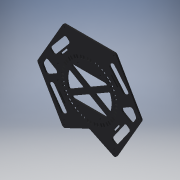
# Autodesk Inventor part: Bottom Plate
Saved by Autodesk Inventor 2017 (Build 210142000, 142)
## iProperties
Created: 2016-10-01
Part Number: Bottom Plate
Material: PVC, Unplasticized
Document SubType Name: Modeling
Designer: James Yelland
Density: 1.29 g/cm^3
Appearance: Smooth - White
Mass: 43.6601 g
Surface Area: 401.333 cm^2
Volume: 33.8451 cm^3
Author: James Yelland
Autodesk Inventor part; units mm, degrees
ref_plane "YZ Plane" through (0, 0, 0) normal (1, 0, 0) x (0, 1, 0)
ref_plane "XZ Plane" through (0, 0, 0) normal (0, 1, 0) x (-1, 0, 0)
ref_plane "XY Plane" through (0, 0, 0) normal (0, 0, 1) x (1, 0, 0)
sketch "Sketch1" plane through (0, 0, 0) normal (0, 1, 0) x (-1, 0, 0)
  line L0 (103.5566, -2.5) -> (54.8095, -86.9325)
  line L1 (-54.8095, -86.9325) -> (-103.5566, -2.5)
  line L2 (-103.5566, 2.5) -> (-53.9434, 88.4327)
  line L3 (-49.6132, 90.9327) -> (49.6132, 90.9327)
  line L4 (53.9434, 88.4327) -> (103.5566, 2.5)
  line L5 (2.1497, -66.9563) -> (48.3297, -88.9468)
  line L6 (-2.1497, -66.9563) -> (-48.3297, -88.9468)
  arc A0 (48.3297, -88.9468) -> (54.8095, -86.9325) centre (50.4794, -84.4325) ccw
  arc A1 (2.1497, -66.9563) -> (-2.1497, -66.9563) centre (0, -71.4706) ccw
  arc A2 (-54.8095, -86.9325) -> (-48.3297, -88.9468) centre (-50.4794, -84.4325) ccw
  arc A3 (-103.5566, 2.5) -> (-103.5566, -2.5) centre (-99.2265, 0) ccw
  arc A4 (-49.6132, 90.9327) -> (-53.9434, 88.4327) centre (-49.6132, 85.9327) ccw
  arc A5 (53.9434, 88.4327) -> (49.6132, 90.9327) centre (49.6132, 85.9327) ccw
  arc A6 (103.5566, -2.5) -> (103.5566, 2.5) centre (99.2265, 0) ccw
  circle A7 centre (49.6132, 85.9327) radius 1.6
  circle A8 centre (-49.6132, 85.9327) radius 1.6
  circle A9 centre (-99.2265, 0) radius 1.6
  circle A10 centre (99.2265, 0) radius 1.6
  arc A11 (-88.75, -10.8253) -> (-81.9199, -12.6554) centre (-84.4199, -8.3253) ccw
  arc A12 (-93.5566, 2.5) -> (-93.5566, -2.5) centre (-89.2265, 0) ccw
  arc A13 (81.9199, -12.6554) -> (88.75, -10.8253) centre (84.4199, -8.3253) ccw
  arc A14 (93.5566, -2.5) -> (93.5566, 2.5) centre (89.2265, 0) ccw
  line L7 (1.5, -53.75) -> (1.5, -56.75)
  line L8 (1.5, -56.75) -> (4.5, -56.75)
  line L9 (4.5, -56.75) -> (4.5, -50.75)
  line L10 (4.5, -50.75) -> (1.5, -50.75)
  line L11 (1.5, -50.75) -> (1.5, -53.75)
  line L12 (-1.5, -53.75) -> (-1.5, -56.75)
  line L13 (-1.5, -56.75) -> (-4.5, -56.75)
  line L14 (-1.5, -53.75) -> (-1.5, -53.75)
  line L15 (-1.5, -53.75) -> (-1.5, -50.75)
  line L16 (-1.5, -50.75) -> (-4.5, -50.75)
  line L17 (-4.5, -56.75) -> (-4.5, -50.75)
  line L18 (15.3604, -51.5303) -> (16.1369, -54.4281)
  line L19 (16.1369, -54.4281) -> (19.0346, -53.6516)
  line L20 (19.0346, -53.6516) -> (17.4817, -47.856)
  line L21 (17.4817, -47.856) -> (14.584, -48.6325)
  line L22 (14.584, -48.6325) -> (15.3604, -51.5303)
  line L23 (12.4626, -52.3067) -> (13.2391, -55.2045)
  line L24 (13.2391, -55.2045) -> (10.3413, -55.981)
  line L25 (12.4626, -52.3067) -> (11.6862, -49.409)
  line L26 (11.6862, -49.409) -> (8.7884, -50.1854)
  line L27 (10.3413, -55.981) -> (8.7884, -50.1854)
  line L28 (28.174, -45.7989) -> (29.674, -48.3969)
  line L29 (29.674, -48.3969) -> (32.2721, -46.8969)
  line L30 (32.2721, -46.8969) -> (29.2721, -41.7008)
  line L31 (29.2721, -41.7008) -> (26.674, -43.2008)
  line L32 (26.674, -43.2008) -> (28.174, -45.7989)
  line L33 (25.576, -47.2989) -> (27.076, -49.8969)
  line L34 (27.076, -49.8969) -> (24.4779, -51.3969)
  line L35 (25.576, -47.2989) -> (24.076, -44.7008)
  line L36 (24.076, -44.7008) -> (21.4779, -46.2008)
  line L37 (24.4779, -51.3969) -> (21.4779, -46.2008)
  line L38 (39.0676, -36.9463) -> (41.189, -39.0676)
  line L39 (41.189, -39.0676) -> (43.3103, -36.9463)
  line L40 (43.3103, -36.9463) -> (39.0676, -32.7037)
  line L41 (39.0676, -32.7037) -> (36.9463, -34.825)
  line L42 (36.9463, -34.825) -> (39.0676, -36.9463)
  line L43 (36.9463, -39.0676) -> (39.0676, -41.189)
  line L44 (39.0676, -41.189) -> (36.9463, -43.3103)
  line L45 (36.9463, -39.0676) -> (34.825, -36.9463)
  line L46 (34.825, -36.9463) -> (32.7037, -39.0676)
  line L47 (36.9463, -43.3103) -> (32.7037, -39.0676)
  line L48 (47.2989, -25.576) -> (49.8969, -27.076)
  line L49 (49.8969, -27.076) -> (51.3969, -24.4779)
  line L50 (51.3969, -24.4779) -> (46.2008, -21.4779)
  line L51 (46.2008, -21.4779) -> (44.7008, -24.076)
  line L52 (44.7008, -24.076) -> (47.2989, -25.576)
  line L53 (45.7989, -28.174) -> (48.3969, -29.674)
  line L54 (48.3969, -29.674) -> (46.8969, -32.2721)
  line L55 (45.7989, -28.174) -> (43.2008, -26.674)
  line L56 (43.2008, -26.674) -> (41.7008, -29.2721)
  line L57 (46.8969, -32.2721) -> (41.7008, -29.2721)
  line L58 (52.3067, -12.4626) -> (55.2045, -13.2391)
  line L59 (55.2045, -13.2391) -> (55.981, -10.3413)
  line L60 (55.981, -10.3413) -> (50.1854, -8.7884)
  line L61 (50.1854, -8.7884) -> (49.409, -11.6862)
  line L62 (49.409, -11.6862) -> (52.3067, -12.4626)
  line L63 (51.5303, -15.3604) -> (54.4281, -16.1369)
  line L64 (54.4281, -16.1369) -> (53.6516, -19.0346)
  line L65 (51.5303, -15.3604) -> (48.6325, -14.584)
  line L66 (48.6325, -14.584) -> (47.856, -17.4817)
  line L67 (53.6516, -19.0346) -> (47.856, -17.4817)
  line L68 (53.75, 1.5) -> (56.75, 1.5)
  line L69 (56.75, 1.5) -> (56.75, 4.5)
  line L70 (56.75, 4.5) -> (50.75, 4.5)
  line L71 (50.75, 4.5) -> (50.75, 1.5)
  line L72 (50.75, 1.5) -> (53.75, 1.5)
  line L73 (53.75, -1.5) -> (56.75, -1.5)
  line L74 (56.75, -1.5) -> (56.75, -4.5)
  line L75 (53.75, -1.5) -> (50.75, -1.5)
  line L76 (50.75, -1.5) -> (50.75, -4.5)
  line L77 (56.75, -4.5) -> (50.75, -4.5)
  line L78 (51.5303, 15.3604) -> (54.4281, 16.1369)
  line L79 (54.4281, 16.1369) -> (53.6516, 19.0346)
  line L80 (53.6516, 19.0346) -> (47.856, 17.4817)
  line L81 (47.856, 17.4817) -> (48.6325, 14.584)
  line L82 (48.6325, 14.584) -> (51.5303, 15.3604)
  line L83 (52.3067, 12.4626) -> (55.2045, 13.2391)
  line L84 (55.2045, 13.2391) -> (55.981, 10.3413)
  line L85 (52.3067, 12.4626) -> (49.409, 11.6862)
  line L86 (49.409, 11.6862) -> (50.1854, 8.7884)
  line L87 (55.981, 10.3413) -> (50.1854, 8.7884)
  line L88 (45.7989, 28.174) -> (48.3969, 29.674)
  line L89 (48.3969, 29.674) -> (46.8969, 32.2721)
  line L90 (46.8969, 32.2721) -> (41.7008, 29.2721)
  line L91 (41.7008, 29.2721) -> (43.2008, 26.674)
  line L92 (43.2008, 26.674) -> (45.7989, 28.174)
  line L93 (47.2989, 25.576) -> (49.8969, 27.076)
  line L94 (49.8969, 27.076) -> (51.3969, 24.4779)
  line L95 (47.2989, 25.576) -> (44.7008, 24.076)
  line L96 (44.7008, 24.076) -> (46.2008, 21.4779)
  line L97 (51.3969, 24.4779) -> (46.2008, 21.4779)
  line L98 (36.9463, 39.0676) -> (39.0676, 41.189)
  line L99 (39.0676, 41.189) -> (36.9463, 43.3103)
  line L100 (36.9463, 43.3103) -> (32.7037, 39.0676)
  line L101 (32.7037, 39.0676) -> (34.825, 36.9463)
  line L102 (34.825, 36.9463) -> (36.9463, 39.0676)
  line L103 (39.0676, 36.9463) -> (41.189, 39.0676)
  line L104 (41.189, 39.0676) -> (43.3103, 36.9463)
  line L105 (39.0676, 36.9463) -> (36.9463, 34.825)
  line L106 (36.9463, 34.825) -> (39.0676, 32.7037)
  line L107 (43.3103, 36.9463) -> (39.0676, 32.7037)
  line L108 (25.576, 47.2989) -> (27.076, 49.8969)
  line L109 (27.076, 49.8969) -> (24.4779, 51.3969)
  line L110 (24.4779, 51.3969) -> (21.4779, 46.2008)
  line L111 (21.4779, 46.2008) -> (24.076, 44.7008)
  line L112 (24.076, 44.7008) -> (25.576, 47.2989)
  line L113 (28.174, 45.7989) -> (29.674, 48.3969)
  line L114 (29.674, 48.3969) -> (32.2721, 46.8969)
  line L115 (28.174, 45.7989) -> (26.674, 43.2008)
  line L116 (26.674, 43.2008) -> (29.2721, 41.7008)
  line L117 (32.2721, 46.8969) -> (29.2721, 41.7008)
  line L118 (12.4626, 52.3067) -> (13.2391, 55.2045)
  line L119 (13.2391, 55.2045) -> (10.3413, 55.981)
  line L120 (10.3413, 55.981) -> (8.7884, 50.1854)
  line L121 (8.7884, 50.1854) -> (11.6862, 49.409)
  line L122 (11.6862, 49.409) -> (12.4626, 52.3067)
  line L123 (15.3604, 51.5303) -> (16.1369, 54.4281)
  line L124 (16.1369, 54.4281) -> (19.0346, 53.6516)
  line L125 (15.3604, 51.5303) -> (14.584, 48.6325)
  line L126 (14.584, 48.6325) -> (17.4817, 47.856)
  line L127 (19.0346, 53.6516) -> (17.4817, 47.856)
  line L128 (-1.5, 53.75) -> (-1.5, 56.75)
  line L129 (-1.5, 56.75) -> (-4.5, 56.75)
  line L130 (-4.5, 56.75) -> (-4.5, 50.75)
  line L131 (-4.5, 50.75) -> (-1.5, 50.75)
  line L132 (-1.5, 50.75) -> (-1.5, 53.75)
  line L133 (1.5, 53.75) -> (1.5, 56.75)
  line L134 (1.5, 56.75) -> (4.5, 56.75)
  line L135 (1.5, 53.75) -> (1.5, 50.75)
  line L136 (1.5, 50.75) -> (4.5, 50.75)
  line L137 (4.5, 56.75) -> (4.5, 50.75)
  line L138 (-15.3604, 51.5303) -> (-16.1369, 54.4281)
  line L139 (-16.1369, 54.4281) -> (-19.0346, 53.6516)
  line L140 (-19.0346, 53.6516) -> (-17.4817, 47.856)
  line L141 (-17.4817, 47.856) -> (-14.584, 48.6325)
  line L142 (-14.584, 48.6325) -> (-15.3604, 51.5303)
  line L143 (-12.4626, 52.3067) -> (-13.2391, 55.2045)
  line L144 (-13.2391, 55.2045) -> (-10.3413, 55.981)
  line L145 (-12.4626, 52.3067) -> (-11.6862, 49.409)
  line L146 (-11.6862, 49.409) -> (-8.7884, 50.1854)
  line L147 (-10.3413, 55.981) -> (-8.7884, 50.1854)
  line L148 (-28.174, 45.7989) -> (-29.674, 48.3969)
  line L149 (-29.674, 48.3969) -> (-32.2721, 46.8969)
  line L150 (-32.2721, 46.8969) -> (-29.2721, 41.7008)
  line L151 (-29.2721, 41.7008) -> (-26.674, 43.2008)
  line L152 (-26.674, 43.2008) -> (-28.174, 45.7989)
  line L153 (-25.576, 47.2989) -> (-27.076, 49.8969)
  line L154 (-27.076, 49.8969) -> (-24.4779, 51.3969)
  line L155 (-25.576, 47.2989) -> (-24.076, 44.7008)
  line L156 (-24.076, 44.7008) -> (-21.4779, 46.2008)
  line L157 (-24.4779, 51.3969) -> (-21.4779, 46.2008)
  line L158 (-39.0676, 36.9463) -> (-41.189, 39.0676)
  line L159 (-41.189, 39.0676) -> (-43.3103, 36.9463)
  line L160 (-43.3103, 36.9463) -> (-39.0676, 32.7037)
  line L161 (-39.0676, 32.7037) -> (-36.9463, 34.825)
  line L162 (-36.9463, 34.825) -> (-39.0676, 36.9463)
  line L163 (-36.9463, 39.0676) -> (-39.0676, 41.189)
  line L164 (-39.0676, 41.189) -> (-36.9463, 43.3103)
  line L165 (-36.9463, 39.0676) -> (-34.825, 36.9463)
  line L166 (-34.825, 36.9463) -> (-32.7037, 39.0676)
  line L167 (-36.9463, 43.3103) -> (-32.7037, 39.0676)
  line L168 (-47.2989, 25.576) -> (-49.8969, 27.076)
  line L169 (-49.8969, 27.076) -> (-51.3969, 24.4779)
  line L170 (-51.3969, 24.4779) -> (-46.2008, 21.4779)
  line L171 (-46.2008, 21.4779) -> (-44.7008, 24.076)
  line L172 (-44.7008, 24.076) -> (-47.2989, 25.576)
  line L173 (-45.7989, 28.174) -> (-48.3969, 29.674)
  line L174 (-48.3969, 29.674) -> (-46.8969, 32.2721)
  line L175 (-45.7989, 28.174) -> (-43.2008, 26.674)
  line L176 (-43.2008, 26.674) -> (-41.7008, 29.2721)
  line L177 (-46.8969, 32.2721) -> (-41.7008, 29.2721)
  line L178 (-52.3067, 12.4626) -> (-55.2045, 13.2391)
  line L179 (-55.2045, 13.2391) -> (-55.981, 10.3413)
  line L180 (-55.981, 10.3413) -> (-50.1854, 8.7884)
  line L181 (-50.1854, 8.7884) -> (-49.409, 11.6862)
  line L182 (-49.409, 11.6862) -> (-52.3067, 12.4626)
  line L183 (-51.5303, 15.3604) -> (-54.4281, 16.1369)
  line L184 (-54.4281, 16.1369) -> (-53.6516, 19.0346)
  line L185 (-51.5303, 15.3604) -> (-48.6325, 14.584)
  line L186 (-48.6325, 14.584) -> (-47.856, 17.4817)
  line L187 (-53.6516, 19.0346) -> (-47.856, 17.4817)
  line L188 (-53.75, -1.5) -> (-56.75, -1.5)
  line L189 (-56.75, -1.5) -> (-56.75, -4.5)
  line L190 (-56.75, -4.5) -> (-50.75, -4.5)
  line L191 (-50.75, -4.5) -> (-50.75, -1.5)
  line L192 (-50.75, -1.5) -> (-53.75, -1.5)
  line L193 (-53.75, 1.5) -> (-56.75, 1.5)
  line L194 (-56.75, 1.5) -> (-56.75, 4.5)
  line L195 (-53.75, 1.5) -> (-50.75, 1.5)
  line L196 (-50.75, 1.5) -> (-50.75, 4.5)
  line L197 (-56.75, 4.5) -> (-50.75, 4.5)
  line L198 (-51.5303, -15.3604) -> (-54.4281, -16.1369)
  line L199 (-54.4281, -16.1369) -> (-53.6516, -19.0346)
  line L200 (-53.6516, -19.0346) -> (-47.856, -17.4817)
  line L201 (-47.856, -17.4817) -> (-48.6325, -14.584)
  line L202 (-48.6325, -14.584) -> (-51.5303, -15.3604)
  line L203 (-52.3067, -12.4626) -> (-55.2045, -13.2391)
  line L204 (-55.2045, -13.2391) -> (-55.981, -10.3413)
  line L205 (-52.3067, -12.4626) -> (-49.409, -11.6862)
  line L206 (-49.409, -11.6862) -> (-50.1854, -8.7884)
  line L207 (-55.981, -10.3413) -> (-50.1854, -8.7884)
  line L208 (-45.7989, -28.174) -> (-48.3969, -29.674)
  line L209 (-48.3969, -29.674) -> (-46.8969, -32.2721)
  line L210 (-46.8969, -32.2721) -> (-41.7008, -29.2721)
  line L211 (-41.7008, -29.2721) -> (-43.2008, -26.674)
  line L212 (-43.2008, -26.674) -> (-45.7989, -28.174)
  line L213 (-47.2989, -25.576) -> (-49.8969, -27.076)
  line L214 (-49.8969, -27.076) -> (-51.3969, -24.4779)
  line L215 (-47.2989, -25.576) -> (-44.7008, -24.076)
  line L216 (-44.7008, -24.076) -> (-46.2008, -21.4779)
  line L217 (-51.3969, -24.4779) -> (-46.2008, -21.4779)
  line L218 (-36.9463, -39.0676) -> (-39.0676, -41.189)
  line L219 (-39.0676, -41.189) -> (-36.9463, -43.3103)
  line L220 (-36.9463, -43.3103) -> (-32.7037, -39.0676)
  line L221 (-32.7037, -39.0676) -> (-34.825, -36.9463)
  line L222 (-34.825, -36.9463) -> (-36.9463, -39.0676)
  line L223 (-39.0676, -36.9463) -> (-41.189, -39.0676)
  line L224 (-41.189, -39.0676) -> (-43.3103, -36.9463)
  line L225 (-39.0676, -36.9463) -> (-36.9463, -34.825)
  line L226 (-36.9463, -34.825) -> (-39.0676, -32.7037)
  line L227 (-43.3103, -36.9463) -> (-39.0676, -32.7037)
  line L228 (-25.576, -47.2989) -> (-27.076, -49.8969)
  line L229 (-27.076, -49.8969) -> (-24.4779, -51.3969)
  line L230 (-24.4779, -51.3969) -> (-21.4779, -46.2008)
  line L231 (-21.4779, -46.2008) -> (-24.076, -44.7008)
  line L232 (-24.076, -44.7008) -> (-25.576, -47.2989)
  line L233 (-28.174, -45.7989) -> (-29.674, -48.3969)
  line L234 (-29.674, -48.3969) -> (-32.2721, -46.8969)
  line L235 (-28.174, -45.7989) -> (-26.674, -43.2008)
  line L236 (-26.674, -43.2008) -> (-29.2721, -41.7008)
  line L237 (-32.2721, -46.8969) -> (-29.2721, -41.7008)
  line L238 (-12.4626, -52.3067) -> (-13.2391, -55.2045)
  line L239 (-13.2391, -55.2045) -> (-10.3413, -55.981)
  line L240 (-10.3413, -55.981) -> (-8.7884, -50.1854)
  line L241 (-8.7884, -50.1854) -> (-11.6862, -49.409)
  line L242 (-11.6862, -49.409) -> (-12.4626, -52.3067)
  line L243 (-15.3604, -51.5303) -> (-16.1369, -54.4281)
  line L244 (-16.1369, -54.4281) -> (-19.0346, -53.6516)
  line L245 (-15.3604, -51.5303) -> (-14.584, -48.6325)
  line L246 (-14.584, -48.6325) -> (-17.4817, -47.856)
  line L247 (-19.0346, -53.6516) -> (-17.4817, -47.856)
  arc A15 (-81.9199, 12.6554) -> (-88.75, 10.8253) centre (-84.4199, 8.3253) ccw
  arc A16 (50.7976, 70.0378) -> (45.1623, 70.5308) centre (47.7335, 67.4666) ccw
  line L248 (45.1623, 70.5308) -> (41.3321, 67.3169)
  arc A17 (41.3321, 67.3169) -> (40.8391, 61.6815) centre (43.9032, 64.2527) ccw
  line L249 (64.2962, 53.9509) -> (50.7976, 70.0378)
  line L250 (40.8391, 61.6815) -> (67.8361, 29.5077)
  line L251 (64.2962, 53.9509) -> (77.7947, 37.8639)
  arc A18 (77.3017, 32.2286) -> (77.7947, 37.8639) centre (74.7305, 35.2928) ccw
  line L252 (73.4714, 29.0147) -> (77.3017, 32.2286)
  arc A19 (67.8361, 29.5077) -> (73.4714, 29.0147) centre (70.9003, 32.0789) ccw
  arc A20 (88.75, 10.8253) -> (81.9199, 12.6554) centre (84.4199, 8.3253) ccw
  arc A21 (67.5, 4.3301) -> (67.5, -4.3301) centre (70, 0) ccw
  arc A22 (-67.5, -4.3301) -> (-67.5, 4.3301) centre (-70, 0) ccw
  line L253 (-67.5, -4.3301) -> (-81.9199, -12.6554)
  line L254 (-88.75, -10.8253) -> (-93.5566, -2.5)
  line L255 (-93.5566, 2.5) -> (-88.75, 10.8253)
  line L256 (-81.9199, 12.6554) -> (-67.5, 4.3301)
  line L257 (81.9199, 12.6554) -> (67.5, 4.3301)
  line L258 (67.5, -4.3301) -> (81.9199, -12.6554)
  line L259 (88.75, -10.8253) -> (93.5566, -2.5)
  line L260 (93.5566, 2.5) -> (88.75, 10.8253)
  line L261 (0, 30) -> (-31.225, 30)
  line L262 (0, 30) -> (31.225, 30)
  line L263 (0, -30) -> (-31.225, -30)
  line L264 (0, -30) -> (31.225, -30)
  arc A23 (42.1141, -15.8557) -> (42.1141, 15.8557) centre (0, 0) ccw
  arc A24 (-42.1141, 15.8558) -> (-42.1141, -15.8558) centre (0, 0) ccw
  arc A25 (34.525, 28.7563) -> (31.225, 30) centre (31.225, 25) ccw
  arc A26 (-31.225, 30) -> (-34.525, 28.7563) centre (-31.225, 25) ccw
  arc A27 (-34.525, -28.7563) -> (-31.225, -30) centre (-31.225, -25) ccw
  arc A28 (31.225, -30) -> (34.525, -28.7563) centre (31.225, -25) ccw
  circle A29 centre (22.6343, 38) radius 1.6
  circle A30 centre (-22.6343, 38) radius 1.6
  circle A31 centre (-22.6343, -38) radius 1.6
  circle A32 centre (22.6343, -38) radius 1.6
  line L265 (54.3376, 45.5946) -> (57.5515, 41.7644)
  line L266 (39.2424, -16.8831) -> (13, -1.7321)
  line L267 (39.2424, 16.8831) -> (13, 1.7321)
  line L268 (34.205, 25.5218) -> (1, 6.3509)
  line L269 (-1, 6.3509) -> (-34.205, 25.5218)
  line L270 (-39.2423, 16.8832) -> (-12.9998, 1.7321)
  line L271 (-12.9998, -1.7321) -> (-39.2423, -16.8832)
  line L272 (-34.205, -25.5218) -> (-1, -6.3509)
  line L273 (1, -6.3509) -> (34.205, -25.5218)
  arc A33 (-1, 6.3509) -> (1, 6.3509) centre (0, 8.0829) ccw
  arc A34 (-12.9998, -1.7321) -> (-12.9998, 1.7321) centre (-13.9998, 0) ccw
  arc A35 (1, -6.3509) -> (-1, -6.3509) centre (0, -8.0829) ccw
  arc A36 (13, 1.7321) -> (13, -1.7321) centre (14, 0) ccw
  arc A37 (39.2424, -16.8831) -> (42.1141, -15.8557) centre (40.2424, -15.151) ccw
  arc A38 (34.525, -28.7563) -> (34.205, -25.5218) centre (33.205, -27.2538) ccw
  arc A39 (-42.1141, -15.8558) -> (-39.2423, -16.8832) centre (-40.2423, -15.1511) ccw
  arc A40 (-34.205, -25.5218) -> (-34.525, -28.7563) centre (-33.205, -27.2538) ccw
  arc A41 (-39.2423, 16.8832) -> (-42.1141, 15.8558) centre (-40.2423, 15.1511) ccw
  arc A42 (-34.525, 28.7563) -> (-34.205, 25.5218) centre (-33.205, 27.2538) ccw
  arc A43 (42.1141, 15.8557) -> (39.2424, 16.8831) centre (40.2424, 15.151) ccw
  arc A44 (34.205, 25.5218) -> (34.525, 28.7563) centre (33.205, 27.2538) ccw
  circle A45 centre (50.4794, -84.4325) radius 1.45
  circle A46 centre (50.4794, -76.4325) radius 1.45
  circle A47 centre (-50.4794, -84.4325) radius 1.45
  circle A48 centre (-50.4794, -76.4325) radius 1.45
  line L274 (49.7796, 41.77) -> (43.3517, 49.4305)
  line L275 (43.3517, 49.4305) -> (45.6499, 51.3589)
  line L276 (45.6499, 51.3589) -> (58.5056, 36.038)
  line L277 (58.5056, 36.038) -> (56.2075, 34.1096)
  line L278 (56.2075, 34.1096) -> (49.7796, 41.77)
  arc A49 (75.7207, -22.5008) -> (70.1497, -23.4831) centre (73.4264, -25.7774) ccw
  arc A50 (80.7987, -30.9396) -> (79.8164, -25.3687) centre (77.5221, -28.6453) ccw
  line L279 (75.7207, -22.5008) -> (79.8164, -25.3687)
  arc A51 (51.1376, -66.3263) -> (56.7085, -65.344) centre (53.4319, -63.0497) ccw
  line L280 (51.1376, -66.3263) -> (47.0419, -63.4584)
  arc A52 (46.0596, -57.8875) -> (47.0419, -63.4584) centre (49.3362, -60.1818) ccw
  line L281 (68.7536, -48.1418) -> (56.7085, -65.344)
  line L282 (68.7536, -48.1418) -> (80.7987, -30.9396)
  line L283 (46.0596, -57.8875) -> (70.1497, -23.4831)
  line L284 (58.1046, -40.6853) -> (60.9725, -36.5895)
  line L285 (53.2307, -37.2725) -> (47.4949, -45.464)
  line L286 (47.4949, -45.464) -> (49.9524, -47.1848)
  line L287 (49.9524, -47.1848) -> (61.4239, -30.8017)
  line L288 (61.4239, -30.8017) -> (58.9665, -29.081)
  line L289 (58.9665, -29.081) -> (53.2307, -37.2725)
  arc A53 (-73.4714, 29.0147) -> (-67.8361, 29.5077) centre (-70.9003, 32.0789) ccw
  arc A54 (-77.7947, 37.8639) -> (-77.3017, 32.2286) centre (-74.7305, 35.2928) ccw
  line L290 (-73.4714, 29.0147) -> (-77.3017, 32.2286)
  arc A55 (-45.1623, 70.5308) -> (-50.7976, 70.0378) centre (-47.7335, 67.4666) ccw
  line L291 (-45.1623, 70.5308) -> (-41.3321, 67.3169)
  arc A56 (-40.8391, 61.6815) -> (-41.3321, 67.3169) centre (-43.9032, 64.2527) ccw
  line L292 (-64.2962, 53.9509) -> (-50.7976, 70.0378)
  line L293 (-64.2962, 53.9509) -> (-77.7947, 37.8639)
  line L294 (-40.8391, 61.6815) -> (-67.8361, 29.5077)
  line L295 (-49.7796, 41.77) -> (-43.3517, 49.4305)
  line L296 (-43.3517, 49.4305) -> (-45.6499, 51.3589)
  line L297 (-45.6499, 51.3589) -> (-58.5056, 36.038)
  line L298 (-58.5056, 36.038) -> (-56.2075, 34.1096)
  line L299 (-56.2075, 34.1096) -> (-49.7796, 41.77)
  arc A57 (-70.1497, -23.4831) -> (-75.7207, -22.5008) centre (-73.4264, -25.7774) ccw
  line L300 (-49.9524, -47.1848) -> (-61.4239, -30.8017)
  line L301 (-61.4239, -30.8017) -> (-58.9665, -29.081)
  line L302 (-46.0596, -57.8875) -> (-70.1497, -23.4831)
  line L303 (-68.7536, -48.1418) -> (-80.7987, -30.9396)
  line L304 (-75.7207, -22.5008) -> (-79.8164, -25.3687)
  arc A58 (-79.8164, -25.3687) -> (-80.7987, -30.9396) centre (-77.5221, -28.6453) ccw
  line L305 (-47.4949, -45.464) -> (-49.9524, -47.1848)
  line L306 (-53.2307, -37.2725) -> (-47.4949, -45.464)
  arc A59 (-56.7085, -65.344) -> (-51.1376, -66.3263) centre (-53.4319, -63.0497) ccw
  line L307 (-68.7536, -48.1418) -> (-56.7085, -65.344)
  line L308 (-51.1376, -66.3263) -> (-47.0419, -63.4584)
  arc A60 (-47.0419, -63.4584) -> (-46.0596, -57.8875) centre (-49.3362, -60.1818) ccw
  line L309 (-58.9665, -29.081) -> (-53.2307, -37.2725)
  circle A61 centre (63.1527, -13.1554) radius 1.6
  circle A62 centre (62.6527, 16.2894) radius 1.6
  point P0 (105, 0)
  point P1 (52.5, -90.9327)
  point P2 (-105, 0)
  point P3 (-52.5, 90.9327)
  point P4 (52.5, 90.9327)
  point P5 (-86.25, -15.1554)
  point P6 (60, 0)
  point P7 (-60, 0)
  point P8 (-60, 0)
  point P9 (38.2679, 64.7457)
  point P10 (48.2265, 73.102)
  point P11 (70.4073, 26.4435)
  point P12 (80.3658, 34.7998)
  point P13 (60, 0)
  point P14 (-33.541, 30)
  point P15 (33.541, 30)
  point P16 (-33.541, -30)
  point P17 (33.541, -30)
  point P18 (41.2298, -18.0305)
  point P19 (41.2298, 18.0305)
  point P20 (-41.2298, 18.0306)
  point P21 (-41.2298, -18.0306)
  point P22 (72.4441, -20.2065)
  point P23 (83.093, -27.663)
  point P24 (43.7652, -61.1641)
  point P25 (54.4142, -68.6206)
  point P26 (-70.4073, 26.4435)
  point P27 (-80.3658, 34.7998)
  point P28 (-38.2679, 64.7457)
  point P29 (-48.2265, 73.102)
  point P30 (-72.4441, -20.2065)
  point P31 (-54.4142, -68.6206)
  point P32 (-83.093, -27.663)
  dimension "d11" = 360
  dimension "d30" = 360
  dimension "d114" = 360
  dimension "d147" = 3.2
  dimension "d148" = 3.2
  constraints: 620 end point, 106 point on circle, 75 point on line, 63 centre point, 5 coincident, 1 midpoint, 1 other
  measures "d147" diameter of A61
  measures "d148" diameter of A62
extrude "Extrusion1" add sketch "Sketch1" along normal blind 3
body "Solid1"
